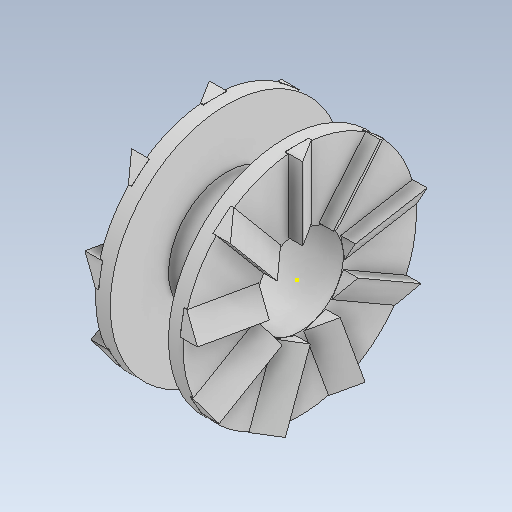
# Autodesk Inventor part: Part10
Saved by Autodesk Inventor 2021 (Build 250183000, 183)
## iProperties
Created: 2022-12-10
Part Number: Part10
Material: Generic
Document SubType Name: Modeling
Designer: user
Density: 1 g/cm^3
Appearance: Default
Author: user
Autodesk Inventor part; units mm, degrees
ref_plane "YZ Plane" through (0, 0, 0) normal (1, 0, 0) x (0, 1, 0)
sketch "Sketch1" plane through (0, 0, 0) normal (0, 0, 1) x (1, 0, 0)
  line L0 (0, 15) -> (0, 40)
  line L1 (0, 40) -> (4, 40)
  line L2 (4, 40) -> (4, 17.6027)
  line L3 (4, 20) -> (24, 20)
  line L4 (24, 17.6027) -> (24, 40)
  line L5 (24, 40) -> (28, 40)
  line L6 (28, 40) -> (28, 15)
  line L7 (30, 0) -> (0, 0)
  line L8 (0, 15) -> (28, 15)
  dimension "d0" = 20
  dimension "d1" = 4
  dimension "d2" = 4
  dimension "d3" = 20
  dimension "d4" = 80
  dimension "d5" = 80
  dimension "d6" = 40
  dimension "d16" = 30
  constraints: 18 end point, 4 perpendicular, 3 horizontal, 2 vertical, 1 point on line
  measures "d0" distance of L3.start L3.end
  measures "d1" distance of L4.end L5.end
  measures "d2" distance of L0.end L1.end
  measures "d3" distance of L4.start L2.end
  measures "d4" diameter of L5 L7
  measures "d5" diameter of L1 L7
  measures "d6" diameter of L3 L7
  measures "d16" diameter of L8 L7
revolve "Revolution1" add sketch "Sketch1" angle 360 about axis through (30, 0, 0) along (-1, 0, 0)
sketch "Sketch3" plane through (28, 0, 0) normal (1, 0, 0) x (0, 0, -1)
  point P0 (0, 0)
sketch "Sketch5" plane through (0, 0, 0) normal (0, 0, 1) x (1, 0, 0)
  point P0 (0, 0)
sketch "Sketch6" plane through (0, 0, 0) normal (0, 0, 1) x (1, 0, 0)
  line L0 (28, -40) -> (28, 40) projected
  line L1 (28, 40) -> (34, 40)
  line L2 (34, 40) -> (34, 15)
  line L3 (34, 15) -> (28, 15)
  line L4 (28, 15) -> (28, 40)
  point P0 (0, 0)
  dimension "d28" = 6
  dimension "d29" = 25
  constraints: 8 end point, 2 parallel, 1 horizontal, 1 perpendicular
  measures "d28" distance of L0.end L1.end
  measures "d29" distance of L1.end L2.end
ref_plane "Work Plane1" through (0, 0, -4) normal (0, 0, 1) x (1, 0, 0)
ref_plane "Work Plane2" through (0, 0, 4) normal (0, 0, 1) x (1, 0, 0)
sketch "Sketch7" plane through (0, 0, 4) normal (0, 0, 1) x (1, 0, 0)
  line L0 (24, 40) -> (28, 40) projected
  line L1 (28, 40) -> (34, 40)
  line L2 (34, 40) -> (34, 15)
  line L3 (34, 15) -> (28, 15)
  line L4 (28, 15) -> (28, 40)
  point P0 (0, 0)
  dimension "d32" = 25
  dimension "d33" = 6
  constraints: 8 end point, 2 parallel, 1 horizontal, 1 perpendicular, 1 point on line
  measures "d32" distance of L1.end L2.end
  measures "d33" distance of L1.start L1.end
sketch "Sketch8" plane through (0, 0, -4) normal (0, 0, 1) x (1, 0, 0)
  line L0 (28, -40) -> (28, 40) projected
  line L1 (28, 40) -> (29, 40)
  line L2 (29, 40) -> (29, 15)
  line L3 (29, 15) -> (28, 15)
  line L4 (28, 15) -> (28, 40)
  point P0 (0, 0)
  dimension "d34" = 1
  dimension "d35" = 25
  constraints: 8 end point, 2 parallel, 1 horizontal, 1 perpendicular
  measures "d34" distance of L2.end L3.end
  measures "d35" distance of L1.end L2.end
loft "Loft1" add profiles "Sketch7", "Sketch8"
pattern_circular "Circular Pattern1" count 9 over 360 about axis through (14, 0, 0) along (1, 0, 0) of "Loft1"
sketch "Sketch9" plane through (28, 15, -4) normal (1, 0, 0) x (0, 0, -1)
  line L0 (-4, 25) -> (0, 25) projected
  line L1 (0, 25) -> (0, 0) projected
  line L2 (0, 25) -> (0, 0)
  arc A0 (5.6418, -3.5093) -> (-4, 0) centre (-4, -15) ccw projected
  line L3 (0, 0) -> (-4, 0)
  arc A1 (5.6418, -3.5093) -> (6.1047, -1.7817) centre (-4, 0) ccw
  line L4 (5.6418, -3.5093) -> (2.5776, -0.9382)
  arc A2 (18.5184, 18.0593) -> (0, 24.7995) centre (-4, -15) ccw projected
  line L5 (2.5776, -0.9382) -> (18.5184, 18.0593)
  arc A3 (18.5184, 18.0593) -> (0, 24.7995) centre (-4, -15) ccw
  constraints: 8 end point, 4 point on circle, 3 tangent, 2 centre point, 2 perpendicular, 1 coincident, 1 vertical
extrude "Extrusion2" add sketch "Sketch9" along normal blind 1
pattern_circular "Circular Pattern2" count 9 over 360 about axis through (14, 0, 0) along (1, 0, 0) of "Extrusion2"
sketch "Sketch11" plane through (0, 0, -4) normal (0, 0, 1) x (1, 0, 0)
  line L0 (0, -40) -> (0, 40) projected
  line L1 (0, 40) -> (-6, 40)
  line L2 (-6, 40) -> (-6, 15)
  line L3 (-6, 15) -> (0, 15)
  line L4 (0, 15) -> (0, 40)
  point P0 (0, 0)
  dimension "d53" = 6
  dimension "d54" = 25
  constraints: 8 end point, 2 parallel, 1 horizontal, 1 perpendicular
  measures "d53" distance of L0.end L1.end
  measures "d54" distance of L1.end L2.end
sketch "Sketch12" plane through (0, 0, 4) normal (0, 0, 1) x (1, 0, 0)
  line L0 (0, -40) -> (0, 40) projected
  line L1 (0, 40) -> (-1, 40)
  line L2 (-1, 40) -> (-1, 15)
  line L3 (-1, 15) -> (0, 15)
  line L4 (0, 15) -> (0, 40)
  point P0 (0, 0)
  dimension "d55" = 1
  dimension "d56" = 25
  constraints: 8 end point, 2 parallel, 1 horizontal, 1 perpendicular
  measures "d55" distance of L0.end L1.end
  measures "d56" distance of L1.end L2.end
loft "Loft2" add profiles "Sketch11", "Sketch12"
pattern_circular "Circular Pattern3" count 9 over 360 about axis through (14, 0, 0) along (1, 0, 0) of "Loft2"
sketch "Sketch13" plane through (0, 15, 4) normal (-1, 0, 0) x (0, 0, 1)
  circle A0 centre (-4, -15) radius 40 projected
  arc A1 (18.5184, 18.0593) -> (0, 24.7995) centre (-4, -15) ccw
  line L0 (0, 25) -> (0, 0) projected
  line L1 (0, 24.7995) -> (0, 0)
  line L2 (0, 0) -> (-4, 0)
  line L3 (0, 0) -> (-8, 0) projected
  line L4 (8.706, -6.0805) -> (2.5776, -0.9382) projected
  line L5 (18.5184, 18.0593) -> (2.5776, -0.9382)
  line L6 (2.5776, -0.9382) -> (5.6418, -3.5093)
  line L7 (8.706, -6.0805) -> (5.6418, -3.5093) projected
  arc A2 (-4, 0) -> (-13.6418, -3.5093) centre (-4, -15) ccw projected
  arc A3 (5.6418, -3.5093) -> (-4, 0) centre (-4, -15) ccw
  point P0 (0, 24.7995)
  constraints: 8 end point, 6 point on circle, 2 centre point, 2 midpoint, 1 perpendicular, 1 vertical
extrude "Extrusion3" add sketch "Sketch13" along normal blind 1 contours L5 L4 A3 L2 L0 A0 picked at (6.4225, 14.9723)
pattern_circular "Circular Pattern4" count 9 over 360 about axis through (14, 0, 0) along (1, 0, 0) of "Extrusion3"
body "Solid1"
